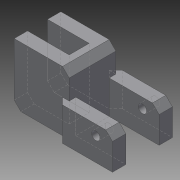
# Autodesk Inventor part: Bottom pully rack
Saved by Autodesk Inventor 2015 (Build 190159000, 159)
## iProperties
Created: 2019-01-17
Part Number: Bottom pully rack
Material: Generic
Document SubType Name: Modeling
Designer: Toby
Density: 1 g/cm^3
Appearance: Default
Author: Toby
Autodesk Inventor part; units mm, degrees
ref_plane "YZ Plane" through (0, 0, 0) normal (1, 0, 0) x (0, 1, 0)
ref_plane "XZ Plane" through (0, 0, 0) normal (0, 1, 0) x (-1, 0, 0)
ref_plane "XY Plane" through (0, 0, 0) normal (0, 0, 1) x (1, 0, 0)
sketch "Sketch1" plane through (0, 0, 0) normal (0, 0, 1) x (1, 0, 0)
  line L0 (-8.218, 3.3953) -> (4.282, 3.3953)
  line L1 (4.282, 3.3953) -> (4.282, -2.6047)
  line L2 (4.282, -2.6047) -> (-8.218, -2.6047)
  line L3 (-8.218, -2.6047) -> (-8.218, 3.3953)
  line L4 (-8.218, 7.3953) -> (8.282, 7.3953)
  line L5 (8.282, 7.3953) -> (8.282, -6.6047)
  line L6 (8.282, -6.6047) -> (-8.218, -6.6047)
  line L7 (-8.218, -6.6047) -> (-8.218, 7.3953)
  point P0 (0, 0)
  dimension "d0" = 12.5
  dimension "d1" = 6
  dimension "d2" = 4
  dimension "d3" = 4
  dimension "d4" = 4
  constraints: 16 end point, 4 parallel, 2 horizontal, 2 perpendicular
  measures "d0" distance of L0.start L0.end
  measures "d1" distance of L0.end L1.end
  measures "d2" distance between parallel lines of L0 L4
  measures "d3" distance between parallel lines of L6 L2
  measures "d4" distance between parallel lines of L5 L1
extrude "Extrusion1" add sketch "Sketch1" along normal blind 18 contours L7 L4 L5 L6 L2 L1 L0
sketch "Sketch2" plane through (8.282, -6.6047, 0) normal (1, 0, 0) x (0, 0, -1)
  line L0 (-10, 12) -> (0, 12)
  line L1 (0, 12) -> (0, 2)
  line L2 (0, 2) -> (-10, 2)
  line L3 (-10, 2) -> (-10, 12)
  line L4 (0, 14) -> (0, 0) projected
  line L5 (0, 14) -> (-18, 14) projected
  line L6 (0, 0) -> (-18, 0) projected
  line L7 (-10, 12) -> (0, 12)
  line L8 (0, 12) -> (0, 16)
  line L9 (0, 16) -> (-10, 16)
  line L10 (-10, 16) -> (-10, 12)
  line L11 (0, 2) -> (-10, 2)
  line L12 (-10, 2) -> (-10, -2)
  line L13 (-10, -2) -> (0, -2)
  line L14 (0, -2) -> (0, 2)
  point P0 (0, 6.6047)
  dimension "d7" = 10
  dimension "d8" = 10
  dimension "d9" = 2
  dimension "d10" = 2
  dimension "d11" = 4
  dimension "d12" = 4
  constraints: 24 end point, 6 parallel, 3 horizontal, 3 perpendicular, 2 collinear, 1 point on line
  measures "d7" distance between parallel lines of L2 L0
  measures "d8" distance of L1.end L2.end
  measures "d9" distance between parallel lines of L5 L0
  measures "d10" distance between parallel lines of L6 L2
  measures "d11" distance of L8.end L7.end
  measures "d12" distance of L12.end L11.end
extrude "Extrusion2" add sketch "Sketch2" along normal blind 15 contours L10 L5 L4 L0 | L2 L4 L6 L12 | L10 L9 L8 L5 | L6 L14 L13 L12
chamfer "Chamfer1" distance 2 angle 45 1 edges at (8.282, -6.6047, 5)
chamfer "Chamfer2" distance 2 angle 45 1 edges at (8.282, 7.3953, 5)
sketch "Sketch3" plane through (23.282, 9.3953, 10) normal (0, 1, 0) x (1, 0, 0)
  line L0 (-15, 0) -> (0, 0) projected
  line L1 (0, 10) -> (0, 0) projected
  circle A0 centre (-5, 3) radius 1.25
  point P0 (-23.282, 10)
  dimension "d21" = 3
  dimension "d22" = 5
  dimension "d23" = 2.5
  constraints: 1 centre point, 1 coincident
  measures "d21" distance from line of L0 point (-5, 3)
  measures "d22" distance from line of L1 point (-5, 3)
  measures "d23" diameter of A0
extrude "Extrusion3" cut sketch "Sketch3" against normal blind 30
chamfer "Chamfer3" distance 2 angle 45 4 edges at (23.282, -6.6047, 10) (23.282, 7.3953, 10) (-8.218, 5.3953, 0) (-8.218, -4.6047, 0)
chamfer "Chamfer4" distance 2 angle 45 1 edges at (8.282, 0.3953, 18)
body "Solid1"
